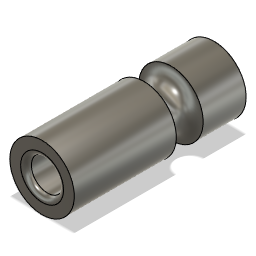
Metal Post and Threaded Rod Assembly (Autodesk Fusion 360 archive; units mm, degrees)
design "Metal Post 1 Inch"
part number: 02-4434
Autodesk Fusion 360 part; units mm, degrees
sketch "Sketch1" plane through (0, 0, 0) normal (0, 1, 0) x (1, 0, 0)
  line L0 (0, 0) -> (0, 25.4)
  line L1 (0, 25.4) -> (4.7625, 25.4)
  line L2 (4.7625, 25.4) -> (4.7625, 19.05)
  line L3 (4.7625, 15.0812) -> (4.7625, 0)
  line L4 (4.7625, 0) -> (0, 0)
  arc A0 (4.7625, 19.05) -> (4.7625, 15.0812) centre (4.7766, 17.0656) ccw
  dimension "d1" = 90
  dimension "d2" = 4.7625
  dimension "d3" = 6.35
  dimension "d4" = 3.9688
  constraint coincident L0.start L4.end
  constraint vertical L0
  constraint perpendicular L1 L2
  constraint perpendicular L0 L4
  measures "d1" angle of L0 L1
  measures "d2" distance of L0.end L1.end
  measures "d3" distance of L1.end L2.end
  measures "d4" distance of L2.end L3.start
sketch "Sketch2" plane through (0, 0, 0) normal (0, 0, 1) x (1, 0, 0)
  circle A0 centre (0, 0) radius 4.7625
  dimension "d5" = 9.525
  constraint coincident A0.centre origin
  measures "d5" diameter of A0
sweep "Sweep1" add profiles "Sketch1" path "Sketch2" along A0 section 1
sketch "Sketch3" plane through (0, 0, -25.4) normal (0, 0, -1) x (-1, 0, 0)
  circle A0 centre (0, 0) radius 4.7625
  circle A1 centre (0, 0) radius 2.3813
  dimension "d12" = 4.7625
  constraint coincident A0.centre A1.centre
  measures "d12" diameter of A1
extrude "Extrude1" cut sketch "Sketch3" against normal blind 25.4 contours A1
fillet "Fillet1" radius 0.3969 1 edges at (2.2201, 0.8611, -25.4)
fillet "Fillet2" radius 0.7937 1 edges at (2.2201, -0.8611, 0)
equation "d2 = ( 3 / 16 ) * 1 in"
equation "d4 = ( 5 / 32 ) * 1 in"
equation "d5 = ( 3 / 8 ) * 1 in"
equation "d12 = ( 3 / 16 ) * 1 in"
equation "d15 = ( 1 / 64 ) * 1 in"
equation "d16 = ( 2 / 64 ) * 1 in"
